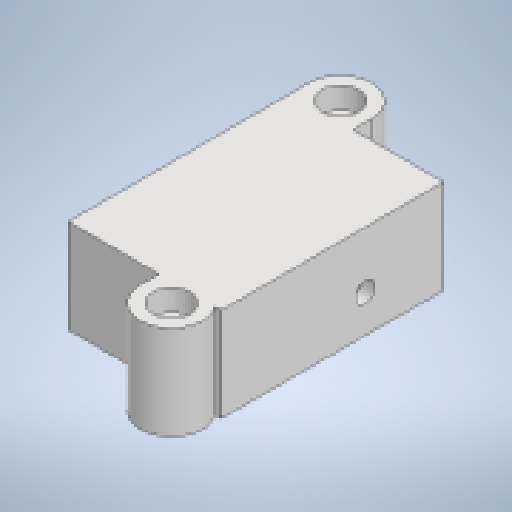
# Autodesk Inventor part: uchwyt_serwa
Saved by Autodesk Inventor 2023 (Build 270158000, 158)
## iProperties
Created: 2024-05-12
Part Number: uchwyt_serwa
Material: Ogólny
Document SubType Name: Modeling
Designer: kamil
Density: 1 g/cm^3
Appearance: Domyślna
Author: kamil
Autodesk Inventor part; units mm, degrees
ref_plane "YZ Plane" through (0, 0, 0) normal (1, 0, 0) x (0, 1, 0)
ref_plane "XZ Plane" through (0, 0, 0) normal (0, 1, 0) x (-1, 0, 0)
ref_plane "XY Plane" through (0, 0, 0) normal (0, 0, 1) x (1, 0, 0)
sketch "Szkic1" plane through (0, 0, 0) normal (0, 1, 0) x (-1, 0, 0)
  line L0 (17, 11.75) -> (0, 11.75)
  line L1 (0, 11.75) -> (0, -11.75)
  line L2 (0, -11.75) -> (17, -11.75)
  line L3 (17, 11.75) -> (17, 17.75)
  line L4 (17, -11.75) -> (17, -17.75)
  line L5 (-5, 17.75) -> (-5, -17.75)
  line L6 (-5, 17.75) -> (17, 17.75)
  line L7 (-5, -17.75) -> (17, -17.75)
  point P0 (0, 0)
  point P1 (0, 0)
  dimension "d0" = 23.5
  dimension "d1" = 17
  dimension "d2" = 6
  dimension "d3" = 6
  dimension "d4" = 5
  constraints: 16 end point, 3 vertical, 2 horizontal, 2 horizontal alignment, 2 perpendicular, 2 vertical alignment, 1 coincident, 1 midpoint, 1 parallel
  measures "d0" distance between parallel lines of L2 L0
  measures "d1" distance of L0.end L0.start
  measures "d2" distance of L0.start L3.end
  measures "d3" distance of L2.end L4.end
  measures "d4" distance between parallel lines of L5 L1
extrude "Wyciągnięcie proste1" add sketch "Szkic1" along normal blind 12
sketch "Szkic2" plane through (0, 12, 0) normal (0, 1, 0) x (1, 0, 0)
  line L0 (5, 17.75) -> (-17, 17.75) projected
  line L1 (-17, 17.75) -> (-17, 11.75) projected
  line L2 (-17, 11.75) -> (0, 11.75) projected
  line L3 (0, 11.75) -> (0, -11.75) projected
  line L4 (0, -11.75) -> (-17, -11.75) projected
  line L5 (-17, -11.75) -> (-17, -17.75) projected
  line L6 (-17, -17.75) -> (5, -17.75) projected
  line L7 (5, -17.75) -> (5, 17.75) projected
  line L8 (-17, -17.75) -> (5, -17.75)
  line L9 (5, -17.75) -> (5, 17.75)
  line L10 (5, 17.75) -> (-17, 17.75)
  line L11 (-17, 17.75) -> (-17, -17.75)
  point P0 (0, 0)
  constraints: 8 end point, 2 parallel, 1 horizontal, 1 perpendicular
extrude "Wyciągnięcie proste2" add sketch "Szkic2" along normal blind 3
sketch "Szkic3" plane through (-17, 0, 11.75) normal (-1, 0, 0) x (0, 0, 1)
  line L0 (0, 0) -> (6, 0) projected
  line L1 (6, 0) -> (6, 15) projected
  line L2 (-29.5, 15) -> (6, 15) projected
  line L3 (-29.5, 0) -> (-29.5, 15) projected
  line L4 (-29.5, 0) -> (-23.5, 0) projected
  line L5 (-23.5, 0) -> (-23.5, 12) projected
  line L6 (-23.5, 12) -> (0, 12) projected
  line L7 (0, 0) -> (0, 12) projected
  line L8 (-23.5, 0) -> (-23.5, 12) projected
  line L9 (-23.5, 12) -> (-28, 12)
  line L10 (-28, 12) -> (-28, 0)
  line L11 (0, 12) -> (4.5, 12)
  line L12 (4.5, 12) -> (4.5, 0)
  point P0 (-11.75, 0)
  dimension "d9" = 1.5
  dimension "d10" = 1.5
  constraints: 8 end point, 2 horizontal, 2 perpendicular, 2 point on line
  measures "d9" distance between parallel lines of L3 L10
  measures "d10" distance between parallel lines of L1 L12
extrude "Wyciągnięcie proste3" add sketch "Szkic3" along normal blind 2.5 contours L12 L11 L6 L9 L10 L4 L3 L2 L1 L0
sketch "Szkic4" plane through (5, 0, -17.75) normal (0, 0, -1) x (-1, 0, 0)
  line L0 (22, 12) -> (22, 0) projected
  line L1 (22, 0) -> (22, 12) projected
  line L2 (12.55, 8.5) -> (12.55, 3.5) construction
  line L3 (10.8, 8.5) -> (10.8, 3.5)
  line L4 (14.3, 3.5) -> (14.3, 8.5)
  arc A0 (14.3, 8.5) -> (10.8, 8.5) centre (12.55, 8.5) ccw
  arc A1 (10.8, 3.5) -> (14.3, 3.5) centre (12.55, 3.5) ccw
  point P0 (5, 0)
  point P1 (12.55, 6)
  point P2 (22, 6)
  dimension "d13" = 3.5
  dimension "d14" = 5
  dimension "d15" = 9.45
  constraints: 8 end point, 4 point on circle, 4 tangent, 2 centre point, 2 midpoint, 1 horizontal alignment, 1 parallel, 1 vertical
  measures "d13" diameter of A1
  measures "d14" distance of L2.start L2.end
  measures "d15" distance from line of L0 point (12.55, 6)
extrude "Wyciągnięcie proste4" cut sketch "Szkic4" against normal up to surface (6 mm away)
sketch "Szkic5" plane through (0, 0, 0) normal (0, -1, 0) x (1, 0, 0)
  line L0 (-9.3, -11.75) -> (-5.8, -11.75) projected
  line L1 (-9.3, -17.75) -> (-9.3, -11.75) projected
  line L2 (-5.8, -17.75) -> (-9.3, -17.75) projected
  line L3 (-5.8, -17.75) -> (-5.8, -11.75) projected
  line L4 (-9.3, -13.75) -> (-5.8, -13.75)
  point P0 (0, 0)
  dimension "d18" = 2
  constraints: 2 end point, 2 point on line, 1 horizontal
  measures "d18" distance between parallel lines of L0 L4
extrude "Wyciągnięcie proste5" cut sketch "Szkic5" against normal blind 5 contours L0 L3 L4 L1
fillet "Zaokrąglenie1" radius 1 1 edges at (-7.55, 1.75, -13.75)
sketch "Szkic6" plane through (0, 0, 0) normal (0, -1, 0) x (1, 0, 0)
  circle A0 centre (0, 20.75) radius 5
  circle A1 centre (-14.5, -20.75) radius 5
  line L0 (5, 17.75) -> (-19.5, 17.75) projected
  line L1 (5, -17.75) -> (-19.5, -17.75) projected
  line L2 (-19.5, -20.75) -> (-19.5, -17.75)
  line L3 (-9.5, -20.75) -> (-9.5, -17.75)
  line L4 (5, 20.75) -> (5, 17.75)
  line L5 (-5, 20.75) -> (-5, 17.75)
  point P0 (0, 0)
  point P1 (-11.25, 17.75)
  point P2 (-11.25, 15.75)
  point P3 (-5.8, -11.75)
  point P4 (5, 20.75)
  point P5 (4, 17.75)
  point P6 (-4, 17.75)
  point P7 (-10.5, -17.75)
  point P8 (-18.5, -17.75)
  dimension "d22" = 10
  dimension "d23" = 10
  dimension "d25" = 2
  dimension "d26" = 3
  constraints: 8 end point, 2 perpendicular, 2 point on circle, 1 centre point, 1 point on line, 1 vertical alignment, 5 other
  measures "d23" diameter of A1
  measures "d25" distance of point (-11.25, 15.75) point (-11.25, 17.75)
  measures "d26" distance from line of L1 A1.centre
extrude "Wyciągnięcie proste6" add sketch "Szkic6" against normal up to surface (15 mm away) contours A0 L0 | A0 L0 L5 | A1 L1 | L2 L1 A1 | A1 L1 L3 picked at (-0.2009, 20.4045) picked at (-14.7009, -20.4045)
sketch "Szkic8" plane through (0, 0, -11.75) normal (-1, 0, 0) x (0, 0, 1)
  circle A0 centre (6.5, 6) radius 0.75 projected
  circle A1 centre (6.5, 6) radius 2.85
  line L0 (8.1454, 8.85) -> (9.7909, 6)
  line L1 (9.7909, 6) -> (8.1454, 3.15)
  line L2 (8.1454, 3.15) -> (4.8546, 3.15)
  line L3 (4.8546, 3.15) -> (3.2091, 6)
  line L4 (3.2091, 6) -> (4.8546, 8.85)
  line L5 (4.8546, 8.85) -> (8.1454, 8.85)
  point P0 (11.75, 0)
  point P1 (6.5, 8.85)
  dimension "d40" = 5.7
  constraints: 12 end point, 2 coincident, 1 midpoint, 1 vertical alignment, 15 other
extrude "Wyciągnięcie proste7" cut sketch "Szkic8" against normal blind 3 contours A0 | A1 | A1 L0 L1 | A1 L5 L0 | L1 L2 A1 | A1 L4 L5 | L2 L3 A1 | A1 L3 L4
sketch "Szkic9" plane through (3, 0, -11.75) normal (-1, 0, 0) x (0, 0, 1)
  circle A0 centre (6.5, 6) radius 0.75 projected
  circle A1 centre (6.5, 6) radius 1.6
  point P0 (11.75, 0)
  dimension "d43" = 3.2
  constraints: 1 centre point, 1 coincident
  measures "d43" diameter of A1
extrude "Wyciągnięcie proste8" cut sketch "Szkic9" against normal through all contours A0 | A1
sketch "Szkic10" plane through (0, 15, 0) normal (0, 1, 0) x (1, 0, 0)
  arc A0 (-5, -20.75) -> (4, -17.75) centre (0, -20.75) ccw projected
  arc A1 (-9.5, 20.75) -> (-19.5, 20.75) centre (-14.5, 20.75) ccw projected
  point P0 (0, 0)
  point P1 (-6.25, -20.75)
  point P2 (-5.8, 20.75)
hole "Otwór2" at (0, 15, 20.75) at (-14.5, 15, -20.75) direction (0, -1, 0) diameter 3.2 end through all counterbore diameter 6 counterbore depth 3.4
sketch "Szkic12" plane through (5, 0, -17.75) normal (0, 0, -1) x (-1, 0, 0)
  line L0 (14.5, 0) -> (14.5, 15) projected
  line L1 (0, 15) -> (14.5, 15) projected
  line L2 (0, 0) -> (0, 15) projected
  line L3 (0, 0) -> (14.5, 0) projected
  line L4 (10.8, 3.5) -> (10.8, 8.5) projected
  arc A0 (14.3, 8.5) -> (10.8, 8.5) centre (12.55, 8.5) ccw projected
  line L5 (14.3, 8.5) -> (14.3, 3.5) projected
  arc A1 (10.8, 3.5) -> (14.3, 3.5) centre (12.55, 3.5) ccw projected
  line L6 (10.8, 8.5) -> (14.3, 8.5)
  line L7 (14.3, 8.5) -> (14.3, -0.3326)
  line L8 (14.3, -0.3326) -> (10.8, -0.3326)
  line L9 (10.8, -0.3326) -> (10.8, 8.5)
  point P0 (5, 0)
  point P1 (10.8, 0)
  point P2 (14.3, 0)
  point P3 (14.3, 3.5)
  constraints: 8 end point, 2 parallel, 1 horizontal, 1 perpendicular
extrude "Wyciągnięcie proste9" cut sketch "Szkic12" against normal up to surface (4 mm away) contours L3 L9 A1 L7
